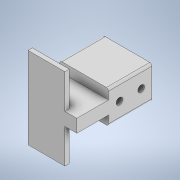
# Autodesk Inventor part: din_lamp_connector
Saved by Autodesk Inventor 2021 (Build 250183000, 183)
## iProperties
Created: 2020-12-10
Part Number: din_lamp_connector
Material: Generic
Document SubType Name: Modeling
Designer: Mateusz
Density: 1 g/cm^3
Appearance: Default
Author: Mateusz
Autodesk Inventor part; units mm, degrees
ref_plane "YZ Plane" through (0, 0, 0) normal (1, 0, 0) x (0, 1, 0)
ref_plane "XZ Plane" through (0, 0, 0) normal (0, 1, 0) x (-1, 0, 0)
ref_plane "XY Plane" through (0, 0, 0) normal (0, 0, 1) x (1, 0, 0)
sketch "Sketch1" plane through (0, 0, 0) normal (1, 0, 0) x (0, 1, 0)
  circle A0 centre (0, -10) radius 3.05
  circle A1 centre (0, -30) radius 3.05
  line L0 (0, 0) -> (6, 0)
  line L1 (6, 0) -> (6, -40)
  line L2 (6, -40) -> (-6, -40)
  line L3 (-6, -40) -> (-6, 0)
  line L4 (-6, 0) -> (0, 0)
  line L5 (6, 0) -> (-6, 0)
  constraints: 12 end point, 3 perpendicular, 2 centre point, 1 collinear, 1 horizontal, 1 point on line
extrude "Extrusion1" add sketch "Sketch1" along normal blind 4
sketch "Sketch2" plane through (0, -6, 0) normal (0, 0, 1) x (1, 0, 0)
  line L0 (0, 12) -> (0, 0) projected
  line L1 (0, 0) -> (4, 0) projected
  line L2 (4, 12) -> (4, 0) projected
  line L3 (0, 12) -> (4, 12) projected
  point P0 (0, 6)
extrude "Extrusion2" add sketch "Sketch2" along normal blind 29.25
sketch "Sketch3" plane through (0, -6, 29.25) normal (0, 0, 1) x (1, 0, 0)
  line L0 (0, 0) -> (0, 12) projected
  line L1 (0, 12) -> (0, 43.7)
  line L2 (0, 0) -> (4, 0) projected
  line L3 (0, 0) -> (0, -31.7)
  line L4 (0, 43.7) -> (34, 43.7)
  line L5 (0, -31.7) -> (34, -31.7)
  line L6 (34, -31.7) -> (34, 43.7)
  line L7 (0, 12) -> (0, 0) projected
  line L8 (0, 0) -> (4, 0) projected
  line L9 (4, 0) -> (4, 12) projected
  line L10 (4, 12) -> (0, 12) projected
  point P0 (0, 6)
  dimension "d12" = 31.7
  dimension "d13" = 31.7
  dimension "d14" = 34
  dimension "d15" = 34
  constraints: 10 end point, 2 horizontal, 2 vertical
  measures "d12" distance of L0.end L1.end
  measures "d13" distance of L0.start L3.end
  measures "d14" distance of L1.end L4.end
  measures "d15" distance of L3.end L5.end
extrude "Extrusion3" add sketch "Sketch3" against normal blind 4 contours L2 L9 L10 L1 L4 L6 L5 L3
sketch "Sketch4" plane through (4, 0, 0) normal (1, 0, 0) x (0, 0, -1)
  line L0 (-25.25, 6) -> (-25.25, -6) projected
  line L1 (40, -6) -> (-25.25, -6) projected
  line L2 (40, -6) -> (40, 6) projected
  line L3 (40, 6) -> (-25.25, 6) projected
  circle A0 centre (10, 0) radius 3.05 projected
  circle A1 centre (30, 0) radius 3.05 projected
  point P0 (0, 0)
extrude "Extrusion4" add sketch "Sketch4" along normal blind 41
sketch "Sketch5" plane through (34, -6, 25.25) normal (0, 0, 1) x (1, 0, 0)
  line L0 (0, 12) -> (0, 0) projected
  line L1 (0, 0) -> (11, 0) projected
  line L2 (11, 12) -> (11, 0) projected
  line L3 (0, 12) -> (11, 12) projected
  point P0 (-34, 6)
extrude "Extrusion5" add sketch "Sketch5" along normal up to surface (4 mm away)
sketch "Sketch6" plane through (0, 6, 25.25) normal (0, 1, 0) x (1, 0, 0)
  line L0 (45, 65.25) -> (45, -4) projected
  line L1 (45, 65.25) -> (45, 25.25)
  line L2 (45, 25.25) -> (0, 25.25)
  line L3 (0, 65.25) -> (45, 65.25) projected
  line L4 (0, 25.25) -> (0, 65.25)
  line L5 (0, 65.25) -> (45, 65.25)
  dimension "d23" = 40
  constraints: 8 end point, 1 perpendicular, 1 point on line
  measures "d23" distance of L0.start L1.end
extrude "Extrusion6" add sketch "Sketch6" along normal blind 9
fillet "Fillet2" radius 2 2 edges at (0, 15, -20) (45, 15, -20)
sketch "Sketch7" plane through (0, -6, 25.25) normal (0, -1, 0) x (1, 0, 0)
  line L0 (45, -25.25) -> (45, -65.25) projected
  line L1 (45, -65.25) -> (45, -25.25)
  line L2 (45, -25.25) -> (0, -25.25) projected
  line L3 (45, -25.25) -> (0, -25.25)
  line L4 (0, -25.25) -> (0, -65.25)
  line L5 (0, -65.25) -> (45, -65.25)
  constraints: 8 end point, 3 perpendicular, 1 collinear
extrude "Extrusion7" add sketch "Sketch7" along normal blind 9
fillet "Fillet3" radius 2 2 edges at (45, -15, -20) (0, -15, -20)
body "Solid1"
